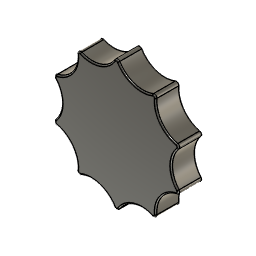
Sugar Jar Cap 2.0 v3 (Autodesk Fusion 360 design; units mm, degrees)
Autodesk Fusion 360 part; units mm, degrees
sketch "Schizzo1" plane through (0, 0, 0) normal (0, 1, 0) x (1, 0, 0)
  circle A0 centre (-56.6885, -32.8751) radius 45
  circle A1 centre (-56.6885, -32.8751) radius 56 construction
  line L0 (-56.6885, -32.8751) -> (-56.6885, -88.8751) construction
  line L1 (-56.6885, -32.8751) -> (-23.7726, -78.1801) construction
  line L2 (-56.6885, -32.8751) -> (-3.4294, -50.1801) construction
  line L3 (-56.6885, -32.8751) -> (-3.4294, -15.5702) construction
  line L4 (-56.6885, -32.8751) -> (-23.7726, 12.4298) construction
  line L5 (-56.6885, -32.8751) -> (-56.6885, 23.1249) construction
  line L6 (-56.6885, -32.8751) -> (-89.6045, 12.4298) construction
  line L7 (-56.6885, -32.8751) -> (-109.9477, -15.5702) construction
  line L8 (-56.6885, -32.8751) -> (-109.9477, -50.1801) construction
  line L9 (-56.6885, -32.8751) -> (-89.6045, -78.1801) construction
  arc A2 (-23.7726, -78.1801) -> (-56.6885, -88.8751) centre (-35.9045, -96.8419) ccw
  arc A3 (-3.4294, -50.1801) -> (-23.7726, -78.1801) centre (-2.2752, -72.4088) ccw
  arc A4 (-3.4294, -15.5702) -> (-3.4294, -50.1801) centre (10.5701, -32.8751) ccw
  arc A5 (-23.7726, 12.4298) -> (-3.4294, -15.5702) centre (-2.2752, 6.6585) ccw
  arc A6 (-56.6885, 23.1249) -> (-23.7726, 12.4298) centre (-35.9045, 31.0916) ccw
  arc A7 (-89.6045, 12.4298) -> (-56.6885, 23.1249) centre (-77.4726, 31.0916) ccw
  arc A8 (-109.9477, -15.5702) -> (-89.6045, 12.4298) centre (-111.1019, 6.6585) ccw
  arc A9 (-109.9477, -50.1801) -> (-109.9477, -15.5702) centre (-123.9472, -32.8751) ccw
  arc A10 (-89.6045, -78.1801) -> (-109.9477, -50.1801) centre (-111.1019, -72.4088) ccw
  arc A11 (-56.6885, -88.8751) -> (-89.6045, -78.1801) centre (-77.4726, -96.8419) ccw
  circle A12 centre (-56.6885, -32.8751) radius 43
  circle A13 centre (-56.6885, -32.8751) radius 42.8
  dimension "d1" = 90
  dimension "d2" = 112
  dimension "d4" = 360
  dimension "d6" = 360
  dimension "d7" = -2
  dimension "d16" = 85.6
  dimension "d25" = 86
  constraint concentric A0 A1
  constraint coincident A0.centre A1.centre
  constraint coincident A1 L0.end
  constraint vertical L0
  constraint tangent A0 A2
  constraint concentric A0 A13
  measures "d1" diameter of A0
  measures "d2" diameter of A1
  measures "d16" diameter of A13
  measures "d25" diameter of A12
extrude "Estrusione3" add sketch "Schizzo1" along normal blind 2 contours A13
extrude "Estrusione4" add sketch "Schizzo1" along normal blind 10 contours A12
extrude "Estrusione1" add sketch "Schizzo1" along normal blind 19 contours A0 | A0 A3 A4 | A0 A4 A5 | A0 A5 A6 | A0 A2 A3 | A0 A6 A7 | A0 A2 A11 | A0 A7 A8 | A0 A10 A11 | A0 A8 A9 | A0 A9 A10
fillet "Raccordo3" radius 2 10 edges at (-3.4294, 9.5, 15.5702) (-23.7726, 9.5, -12.4298) (-56.6885, 9.5, -23.1249) (-89.6045, 9.5, -12.4298) (-109.9477, 9.5, 15.5702) (-109.9477, 9.5, 50.1801) (-89.6045, 9.5, 78.1801) (-56.6885, 9.5, 88.8751) (-23.7726, 9.5, 78.1801) (-3.4294, 9.5, 50.1801)
fillet "Raccordo4" radius 1 20 edges at (-88.1095, 0, 76.1224) (-93.0943, 0, 59.3255) (-107.5288, 0, 49.3941) (-101.6885, 0, 32.8751) (-107.5288, 0, 16.3561) (-93.0943, 0, 6.4248) (-88.1095, 0, -10.3722) (-70.5943, 0, -9.9224) (-56.6885, 0, -20.5815) (-42.7828, 0, -9.9224) (-25.2675, 0, -10.3722) (-20.2828, 0, 6.4248) (-5.8483, 0, 16.3561) (-11.6885, 0, 32.8751) (-5.8483, 0, 49.3941) (-20.2828, 0, 59.3255) (-25.2675, 0, 76.1224) (-42.7828, 0, 75.6727) (-56.6885, 0, 86.3317) (-70.5943, 0, 75.6727)
equation "d16 = 86 mm - 0.4 mm"
